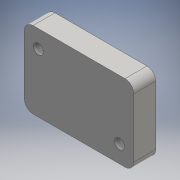
# Autodesk Inventor part: Small Bracket (LHS)
Saved by Autodesk Inventor 2016 (Build 200138000, 138)
## iProperties
Created: 2018-10-20
Part Number: Small Bracket (LHS)
Material: Generic
Document SubType Name: Modeling
Designer: DML
Density: 1 g/cm^3
Appearance: Default
Author: DML
Autodesk Inventor part; units mm, degrees
ref_plane "YZ Plane" through (0, 0, 0) normal (1, 0, 0) x (0, 1, 0)
ref_plane "XZ Plane" through (0, 0, 0) normal (0, 1, 0) x (-1, 0, 0)
ref_plane "XY Plane" through (0, 0, 0) normal (0, 0, 1) x (1, 0, 0)
sketch "Sketch1" plane through (0, 0, 0) normal (0, 1, 0) x (-1, 0, 0)
  line L0 (0, 0) -> (50, 0)
  line L1 (50, 0) -> (50, -35)
  line L2 (50, -35) -> (0, -35)
  line L3 (0, -35) -> (0, 0)
  dimension "d0" = 50
  dimension "d1" = 35
  constraints: 8 end point, 2 parallel, 1 horizontal, 1 perpendicular
  measures "d0" distance of L1.end L2.end
  measures "d1" distance of L0.end L1.end
extrude "Extrusion1" add sketch "Sketch1" along normal blind 10
sketch "Sketch2" plane through (0, 10, 0) normal (0, 1, 0) x (1, 0, 0)
  circle A0 centre (-25, 17.5) radius 11.25
  line L0 (0, 35) -> (-50, 35) projected
  line L1 (-50, 35) -> (-50, 0) projected
  point P0 (0, 0)
  dimension "d4" = 22.5
  dimension "d5" = 17.5
  dimension "d6" = 25
  constraints: 1 centre point
  measures "d4" diameter of A0
  measures "d5" distance from line of L0 A0.centre
  measures "d6" distance from line of L1 A0.centre
extrude "Extrusion2" cut sketch "Sketch2" against normal blind 5
sketch "Sketch3" plane through (0, 10, 0) normal (0, 1, 0) x (1, 0, 0)
  line L0 (-50, 35) -> (-50, 0) projected
  line L1 (-50, 0) -> (0, 0) projected
  line L2 (0, 0) -> (0, 35) projected
  line L3 (0, 35) -> (-50, 35) projected
  point P0 (-43.5, 8)
  point P1 (-6.5, 27)
  dimension "d9" = 6.5
  dimension "d10" = 8
  dimension "d11" = 6.5
  dimension "d12" = 8
  measures "d9" distance from line of L0 point (-43.5, 8)
  measures "d10" distance from line of L1 point (-43.5, 8)
  measures "d11" distance from line of L2 point (-6.5, 27)
  measures "d12" distance from line of L3 point (-6.5, 27)
hole "Hole1" at (-43.5, 10, -8) at (-6.5, 10, -27) direction (0, -1, 0) diameter 4.5 depth 20 tip angle 118 counterbore diameter 8.5 counterbore depth 4
fillet "Fillet1" radius 4 1 edges at (0, 5, 0)
fillet "Fillet2" radius 4 3 edges at (0, 5, -35) (-50, 5, -35) (-50, 5, 0)
body "Solid1"
